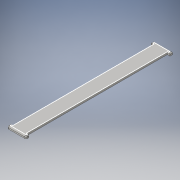
# Autodesk Inventor part: Arm Top
Saved by Autodesk Inventor 2016 (Build 200138000, 138)
## iProperties
Created: 2016-04-25
Part Number: Arm Top
Material: Generic
Document SubType Name: Modeling
Designer: rubenjm
Density: 1 g/cm^3
Appearance: Default
Author: rubenjm
Autodesk Inventor part; units mm, degrees
ref_plane "YZ Plane" through (0, 0, 0) normal (1, 0, 0) x (0, 1, 0)
ref_plane "XZ Plane" through (0, 0, 0) normal (0, 1, 0) x (-1, 0, 0)
ref_plane "XY Plane" through (0, 0, 0) normal (0, 0, 1) x (1, 0, 0)
sketch "Sketch1" plane through (0, 0, 0) normal (0, 1, 0) x (-1, 0, 0)
  line L0 (0, 0) -> (88.9, 0)
  line L1 (88.9, -698.5) -> (0, -698.5)
  line L2 (88.9, 0) -> (76.2, 0) construction
  line L3 (76.2, 0) -> (76.2, -12.7) construction
  line L4 (76.2, -12.7) -> (88.9, -12.7) construction
  line L5 (88.9, -12.7) -> (88.9, 0) construction
  line L6 (0, -349.25) -> (88.9, -349.25) construction
  line L7 (44.45, -698.5) -> (44.45, 0) construction
  line L8 (88.9, -698.5) -> (76.2, -698.5) construction
  line L9 (76.2, -698.5) -> (76.2, -685.8) construction
  line L10 (76.2, -685.8) -> (88.9, -685.8) construction
  line L11 (88.9, -685.8) -> (88.9, -698.5) construction
  line L12 (0, 0) -> (12.7, 0) construction
  line L13 (12.7, 0) -> (12.7, -12.7) construction
  line L14 (12.7, -12.7) -> (0, -12.7) construction
  line L15 (0, -12.7) -> (0, 0) construction
  line L16 (0, -698.5) -> (12.7, -698.5) construction
  line L17 (12.7, -698.5) -> (12.7, -685.8) construction
  line L18 (12.7, -685.8) -> (0, -685.8) construction
  line L19 (0, -685.8) -> (0, -698.5) construction
  line L20 (88.9, -12.7) -> (76.2, -12.7)
  line L21 (76.2, -12.7) -> (76.2, -685.8)
  line L22 (76.2, -685.8) -> (88.9, -685.8)
  line L23 (12.7, -685.8) -> (0, -685.8)
  line L24 (0, -12.7) -> (12.7, -12.7)
  line L25 (12.7, -12.7) -> (12.7, -685.8)
  line L26 (0, -698.5) -> (0, -685.8)
  line L27 (0, -12.7) -> (0, 0)
  line L28 (88.9, 0) -> (88.9, -12.7)
  line L29 (88.9, -685.8) -> (88.9, -698.5)
  dimension "d0" = 88.9
  dimension "d1" = 698.5
  dimension "d2" = 12.7
  dimension "d3" = 12.7
  constraints: 60 end point, 9 parallel, 9 symmetric about line, 4 horizontal, 4 perpendicular, 2 midpoint
  measures "d0" distance of L1.start L1.end
  measures "d1" distance of L0.end L1.start
  measures "d2" distance of L4.end L3.end
  measures "d3" distance of L3.end L2.end
extrude "Extrusion1" add sketch "Sketch1" along normal blind 12.7
fillet "Fillet1" radius 6.35 1 edges at (-44.45, 12.7, 0)
fillet "Fillet2" radius 6.35 9 edges at (0, 10.8401, -1.8599) (0, 3.175, 0) (0, 12.7, -9.525) (-88.9, 10.8401, -1.8599) (-88.9, 3.175, 0) (-88.9, 12.7, -9.525) (-44.45, 12.7, -698.5) (0, 12.7, -692.15) (-88.9, 12.7, -692.15)
body "Solid1"
